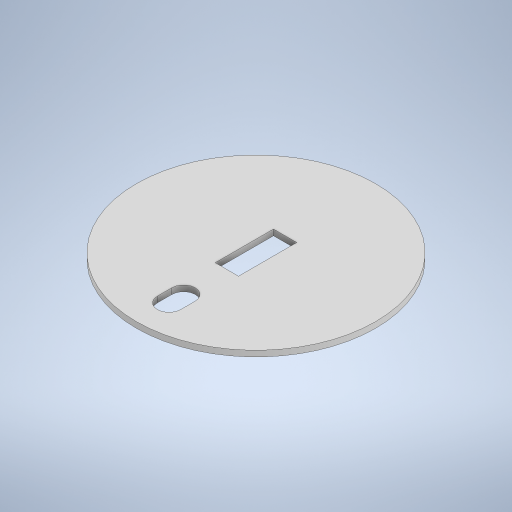
# Autodesk Inventor part: Tic-Tac Baseplate v2
Saved by Autodesk Inventor 2023 (Build 270158000, 158)
## iProperties
Created: 2022-10-31
Part Number: Tic-Tac Baseplate v2
Material: Generic
Document SubType Name: Modeling
Designer: Raker
Density: 1 g/cm^3
Appearance: Default
Mass: 10.087 g
Surface Area: 107.797 cm^2
Volume: 10.087 cm^3
Author: Raker
Autodesk Inventor part; units mm, degrees
ref_plane "YZ Plane" through (0, 0, 0) normal (1, 0, 0) x (0, 1, 0)
ref_plane "XZ Plane" through (0, 0, 0) normal (0, 1, 0) x (-1, 0, 0)
ref_plane "XY Plane" through (0, 0, 0) normal (0, 0, 1) x (1, 0, 0)
sketch "Sketch1" plane through (0, 0, 0) normal (0, 1, 0) x (-1, 0, 0)
  circle A0 centre (0, 0) radius 41
  line L0 (-4, 10) -> (4, 10)
  line L1 (4, 10) -> (4, -10)
  line L2 (4, -10) -> (-4, -10)
  line L3 (-4, -10) -> (-4, 10)
  line L4 (-4, 10) -> (4, -10) construction
  line L5 (4, 10) -> (-4, -10) construction
  circle A1 centre (0, 0) radius 27.3333 construction
  line L6 (0, 20.8333) -> (0, 33.8333) construction
  line L7 (4, 29.8333) -> (4, 24.8333)
  line L8 (-4, 29.8333) -> (-4, 24.8333)
  arc A2 (2.7505, 27.1946) -> (2.625, 27.3333) centre (0, 24.8333) ccw
  arc A3 (-2.625, 27.3333) -> (-2.7505, 27.1946) centre (0, 24.8333) ccw
  arc A4 (-4, 24.8333) -> (4, 24.8333) centre (0, 24.8333) ccw
  arc A5 (2.51, 27.2178) -> (2.625, 27.3333) centre (0, 29.8333) ccw
  arc A6 (4, 29.8333) -> (-4, 29.8333) centre (0, 29.8333) ccw
  arc A7 (-2.625, 27.3333) -> (-2.51, 27.2178) centre (0, 29.8333) ccw
  point P0 (0, 27.3333)
  point P1 (1.5875, 22.7958)
  dimension "d0" = 8
  dimension "d1" = 20
  dimension "d2" = 82
  dimension "d4" = 54.6667
  dimension "d5" = 13
  dimension "d11" = 4
  constraints: 19 point on circle, 18 end point, 8 centre point, 4 tangent, 3 midpoint, 2 coincident, 2 parallel, 2 vertical, 1 horizontal, 1 perpendicular, 1 point on line, 1 vertical alignment
  measures "d0" distance of L1.end L2.end
  measures "d1" distance of L0.end L1.end
  measures "d2" diameter of A0
  measures "d4" diameter of A1
  measures "d5" distance of L6.start L6.end
  measures "d11" radius of A4
extrude "Extrusion1" add sketch "Sketch1" along normal blind 2
body "Solid1"
